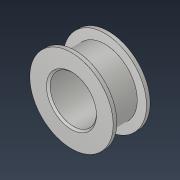
# Autodesk Inventor part: Rolle
Saved by Autodesk Inventor 2022.1 (Build 261234020, 234B)
## iProperties
Part Number: Rolle
Material: Aluminium 6061
Document SubType Name: Modeling
Designer: rYan
Mass: 0.25612 g
Surface Area: 2.90477 cm^2
Volume: 0.0948593 cm^3
Density: 2.7 g/cm^3
Appearance: Aluminium - flach
Author: rYan
Autodesk Inventor part; units mm, degrees
ref_plane "YZ Plane" through (0, 0, 0) normal (1, 0, 0) x (0, 1, 0)
ref_plane "XZ Plane" through (0, 0, 0) normal (0, 1, 0) x (-1, 0, 0)
ref_plane "XY Plane" through (0, 0, 0) normal (0, 0, 1) x (1, 0, 0)
sketch "Skizze1" plane through (0, 0, 0) normal (0, 0, 1) x (1, 0, 0)
  line L0 (0, -2) -> (0, 2)
  line L1 (2.5, 2) -> (2.5, -2)
  line L2 (4.5, -2) -> (4.5, -1.6)
  line L3 (4.5, -1.6) -> (3.5, -1.6)
  line L4 (3.5, -1.6) -> (3.5, 1.6)
  line L5 (3.5, 1.6) -> (4.5, 1.6)
  line L6 (4.5, 1.6) -> (4.5, 2)
  line L7 (-0.9, 0) -> (5.4, 0) projected
  line L8 (4.5, -2) -> (2.5, -2)
  line L9 (4.5, 2) -> (2.5, 2)
  point P0 (0, 0)
  point P1 (0, 0)
  dimension "d0" = 5
  dimension "d3" = 7
  dimension "d4" = 1
  dimension "d6" = 4
  dimension "d8" = 3.2
  constraints: 18 end point, 3 perpendicular, 3 point on line, 2 vertical, 1 coincident, 1 midpoint, 3 other
  measures "d0" diameter of L1 L0
  measures "d3" diameter of L4 L0
  measures "d4" distance between parallel lines of L4 L6
  measures "d6" distance between parallel lines of L8 L9
  measures "d8" distance between parallel lines of L3 L5
revolve "Umdrehung1" add sketch "Skizze1" angle 360 about axis through (0, -2, 0) along (0, 1, 0)
chamfer "Fase2" distance 0.2 angle 45 2 edges at (-2.5, 2, 0) (-2.5, -2, 0)
